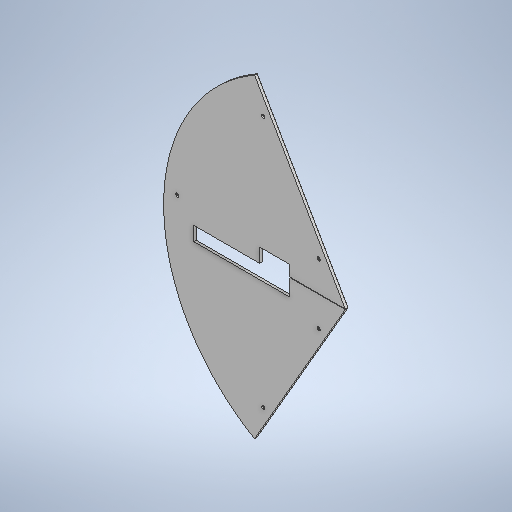
# Autodesk Inventor part: cover
Saved by Autodesk Inventor 2025.1 (Build 291241000, 241)
## iProperties
Created: 2024-11-18
Part Number: cover
Material: Generisch
Document SubType Name: Modeling
Designer: ZOMBULLI
Density: 1 g/cm^3
Appearance: Vorgabe
Author: ZOMBULLI
Autodesk Inventor part; units mm, degrees
ref_plane "YZ Plane" through (0, 0, 0) normal (1, 0, 0) x (0, 1, 0)
ref_plane "XZ Plane" through (0, 0, 0) normal (0, 1, 0) x (-1, 0, 0)
ref_plane "XY Plane" through (0, 0, 0) normal (0, 0, 1) x (1, 0, 0)
sketch "Skizze1" plane through (0, 0, 0) normal (0, 1, 0) x (-1, 0, 0)
  line L0 (0, 0) -> (90, 155.8846)
  line L1 (0, 0) -> (90, -155.8846)
  arc A0 (90, -155.8846) -> (90, 155.8846) centre (0, 0) ccw
  line L2 (216, 0) -> (-36, 0) projected
  dimension "d0" = 360
  dimension "d1" = 120
  dimension "d2" = 60
  constraints: 4 end point, 2 point on circle, 1 centre point, 1 coincident
  measures "d0" diameter of A0
  measures "d1" angle of L1 L0
  measures "d2" angle of L2 L0
extrude "Extrusion1" add sketch "Skizze1" along normal blind 3
fillet "Rundung1" radius 0.5 3 edges at (-45, 3, 77.9423) (-180, 3, 0) (-45, 3, -77.9423)
sketch "Skizze2" plane through (0, 3, 0) normal (0, 1, 0) x (1, 0, 0)
  line L0 (-150, 3) -> (-85, 3)
  line L1 (-55, 3) -> (-55, 17)
  line L2 (-55, 17) -> (-150, 17)
  line L3 (-150, 17) -> (-150, 3)
  line L4 (-227.898, 0) -> (107.3877, 0) projected
  line L5 (-85, 3) -> (-85, -11)
  line L6 (-85, -11) -> (-55, -11)
  line L7 (-55, -11) -> (-55, 3)
  point P0 (0, 0)
  point P1 (-55, 10)
  point P2 (-150, 10)
  dimension "d6" = 14
  dimension "d7" = 95
  dimension "d8" = 17
  dimension "d10" = 150
  dimension "d13" = 30
  dimension "d14" = 14
  constraints: 14 end point, 3 perpendicular, 2 midpoint, 2 parallel, 1 horizontal, 1 vertical
  measures "d6" distance between parallel lines of L2 L0
  measures "d7" distance of point (-55, 10) point (-150, 10)
  measures "d8" distance between parallel lines of L2 L4
  measures "d10" horizontal distance of point (0, 0) point (-150, 10)
  measures "d13" distance of L5.end L6.end
  measures "d14" distance between parallel lines of L0 L6
extrude "Extrusion2" cut sketch "Skizze2" against normal blind 3
fillet "Rundung2" radius 0.5 6 edges at (-102.5, 3, -17) (-117.5, 3, -3) (-150, 3, -10) (-85, 3, 4) (-70, 3, 11) (-55, 3, -3)
sketch "Skizze3" plane through (0, 3, 0) normal (0, 1, 0) x (1, 0, 0)
  line L0 (0, -0.25) -> (-60, -0.25)
  line L1 (-60, -0.25) -> (-60, 0.25)
  line L2 (-60, 0.25) -> (0, 0.25)
  line L3 (0, 0.25) -> (0, -0.25)
  line L4 (-216, 0) -> (36, 0) projected
  point P0 (0, 0)
  point P1 (0, 0)
  dimension "d16" = 0.5
  dimension "d17" = 0.25
  dimension "d18" = 60
  dimension "d19" = 0
  constraints: 8 end point, 2 parallel, 1 horizontal, 1 midpoint, 1 perpendicular
  measures "d16" distance between parallel lines of L2 L0
  measures "d17" distance between parallel lines of L0 L4
  measures "d18" distance between parallel lines of L1 L3
  measures "d19" distance of point (0, 0) point (0, 0)
extrude "Extrusion3" cut sketch "Skizze3" against normal blind 3
sketch "Skizze4" plane through (0, 3, 0) normal (0, 1, 0) x (1, 0, 0)
  circle A0 centre (-81.406, -125) radius 1.65
  circle A1 centre (-26.558, -30) radius 1.65
  circle A2 centre (-166.5, -14.8) radius 1.65
  circle A3 centre (-81.406, 125) radius 1.65
  circle A4 centre (-26.558, 30) radius 1.65
  point P0 (0, 0)
  dimension "d26" = 26.558
  dimension "d27" = 26.558
  dimension "d28" = 3.3
  dimension "d29" = 81.406
  dimension "d30" = 81.406
  dimension "d31" = 14.8
  dimension "d32" = 166.5
  dimension "d33" = 125
  dimension "d34" = 30
  dimension "d35" = 30
  dimension "d36" = 125
  constraints: 5 centre point, 4 equal radius
  measures "d26" horizontal distance of point (0, 0) A1.centre
  measures "d27" horizontal distance of point (0, 0) A4.centre
  measures "d28" diameter of A1
  measures "d29" horizontal distance of A0.centre point (0, 0)
  measures "d30" horizontal distance of point (0, 0) A3.centre
  measures "d31" vertical distance of A2.centre point (0, 0)
  measures "d32" horizontal distance of A2.centre point (0, 0)
  measures "d33" vertical distance of A0.centre point (0, 0)
  measures "d34" vertical distance of point (0, 0) A1.centre
  measures "d35" vertical distance of A4.centre point (0, 0)
  measures "d36" vertical distance of A3.centre point (0, 0)
extrude "Extrusion4" cut sketch "Skizze4" against normal blind 3
chamfer "Fasen1" distance 1.9 angle 45 5 edges at (-83.056, 3, -125) (-28.208, 3, -30) (-28.208, 3, 30) (-83.056, 3, 125) (-168.15, 3, 14.8)
